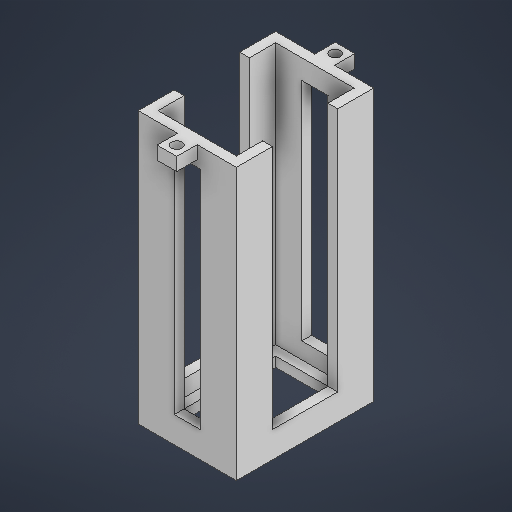
# Autodesk Inventor part: mocowanie-bateria
Saved by Autodesk Inventor 2026.2 (Build 302298010, 298A)
## iProperties
Created: 2026-04-20
Part Number: mocowanie-bateria
Material: Ogólny
Document SubType Name: Modeling
Designer: macie
Density: 1 g/cm^3
Appearance: Domyślna
Author: macie
Autodesk Inventor part; units mm, degrees
ref_plane "YZ Plane" through (0, 0, 0) normal (1, 0, 0) x (0, 1, 0)
ref_plane "XZ Plane" through (0, 0, 0) normal (0, 1, 0) x (-1, 0, 0)
ref_plane "XY Plane" through (0, 0, 0) normal (0, 0, 1) x (1, 0, 0)
sketch "Szkic1" plane through (0, 0, 0) normal (0, 1, 0) x (-1, 0, 0)
  line L0 (12, 18) -> (-12, 18)
  line L1 (-12, 18) -> (-12, -18)
  line L2 (-12, -18) -> (12, -18)
  line L3 (12, -18) -> (12, 18)
  line L4 (12, 18) -> (-12, -18) construction
  line L5 (-12, 18) -> (12, -18) construction
  line L6 (15, 21) -> (-15, 21)
  line L7 (-15, 21) -> (-15, -21)
  line L8 (-15, -21) -> (15, -21)
  line L9 (15, -21) -> (15, 21)
  line L10 (15, 21) -> (-15, -21) construction
  line L11 (-15, 21) -> (15, -21) construction
  line L12 (9, 15) -> (-9, 15)
  line L13 (-9, 15) -> (-9, -15)
  line L14 (-9, -15) -> (9, -15)
  line L15 (9, -15) -> (9, 15)
  line L16 (9, 15) -> (-9, -15) construction
  line L17 (-9, 15) -> (9, -15) construction
  point P0 (0, 0)
  dimension "d0" = 24
  dimension "d1" = 36
  dimension "d2" = 42
  dimension "d3" = 30
  dimension "d4" = 18
  dimension "d5" = 30
  constraints: 36 end point, 6 midpoint, 6 parallel, 3 horizontal, 3 perpendicular
  measures "d0" distance between parallel lines of L1 L3
  measures "d1" distance between parallel lines of L2 L0
  measures "d2" distance between parallel lines of L8 L6
  measures "d3" distance between parallel lines of L7 L9
  measures "d4" distance between parallel lines of L13 L15
  measures "d5" distance between parallel lines of L14 L12
extrude "Wyciągnięcie proste1" add sketch "Szkic1" along normal blind 3 contours L3 L2 L1 L0
extrude "Wyciągnięcie proste2" add sketch "Szkic1" along normal blind 8 contours L9 L8 L7 L6
sketch "Szkic2" plane through (0, 8, 0) normal (0, 1, 0) x (1, 0, 0)
  line L0 (-15, 21) -> (-15, -21) projected
  line L1 (-12, -18) -> (12, -18) projected
  line L2 (-15, -21) -> (-4, -21)
  line L3 (-4, -21) -> (-4, -18)
  line L4 (-4, -18) -> (-15, -18)
  line L5 (-15, -18) -> (-15, -21)
  line L6 (-12, -18) -> (-15, -18)
  line L7 (-15, -18) -> (-15, -10)
  line L8 (-15, -10) -> (-12, -10)
  line L9 (-12, -10) -> (-12, -18)
  line L10 (-15, -21) -> (-15, -10)
  line L11 (0, 0) -> (-18.1992, 0)
  line L12 (-15, 21) -> (-4, 21)
  line L13 (-4, 21) -> (-4, 18)
  line L14 (-4, 18) -> (-15, 18)
  line L15 (-15, 10) -> (-12, 10)
  line L16 (-12, 10) -> (-12, 18)
  line L17 (4, 18) -> (15, 18)
  line L18 (4, 21) -> (4, 18)
  line L19 (15, 21) -> (4, 21)
  line L20 (15, 21) -> (15, 10)
  line L21 (15, 10) -> (12, 10)
  line L22 (12, 10) -> (12, 18)
  line L23 (12, -10) -> (12, -18)
  line L24 (15, -10) -> (12, -10)
  line L25 (4, -18) -> (15, -18)
  line L26 (15, -21) -> (4, -21)
  line L27 (4, -21) -> (4, -18)
  line L28 (15, -21) -> (15, 21) projected
  line L29 (15, -21) -> (15, -10)
  point P0 (-4, -19.5)
  point P1 (4, 19.5)
  dimension "d10" = 11
  dimension "d11" = 8
  dimension "d12" = 18.1992
  dimension "d15" = 360
  constraints: 54 end point, 6 symmetric about line, 4 parallel, 3 horizontal, 2 collinear, 2 perpendicular, 2 point on line, 1 midpoint, 53 other
  measures "d10" distance from line of L0 point (-4, -19.5)
  measures "d11" distance between parallel lines of L8 L4
  measures "d12" distance of L11.start L11.end
extrude "Wyciągnięcie proste3" add sketch "Szkic2" along normal blind 75
sketch "Szkic3" plane through (-4, 8, 21) normal (1, 0, 0) x (0, 0, -1)
  line L0 (0, 75) -> (3, 75) projected
  line L1 (3, -5) -> (3, 75) projected
  line L2 (0, 75) -> (3, 75)
  line L3 (3, 75) -> (3, 69)
  line L4 (3, 69) -> (0, 69)
  line L5 (0, 69) -> (0, 75)
  line L6 (21, 73.1209) -> (21, -14.9491)
  line L7 (0, -8) -> (0, 75) projected
  line L8 (42, 75) -> (39, 75)
  line L9 (39, -5) -> (39, 75)
  line L10 (39, 69) -> (42, 69)
  line L11 (42, 69) -> (42, 75)
  point P0 (21, -8)
  dimension "d19" = 6
  dimension "d20" = 88.0699
  dimension "d21" = 21
  constraints: 18 end point, 5 symmetric about line, 2 parallel, 2 point on line, 1 horizontal, 1 perpendicular, 1 vertical
  measures "d19" distance between parallel lines of L4 L0
  measures "d20" distance of L6.end L6.start
  measures "d21" distance between parallel lines of L7 L6
extrude "Wyciągnięcie proste4" add sketch "Szkic3" along normal blind 9
sketch "Szkic7" plane through (-15, 0, 21) normal (0, 0, 1) x (1, 0, 0)
  line L0 (27, 83) -> (3, 83) projected
  line L1 (12, 83) -> (18, 83)
  line L2 (18, 83) -> (18, 79)
  line L3 (18, 79) -> (12, 79)
  line L4 (12, 79) -> (12, 83)
  line L5 (19, 8) -> (19, 77) projected
  point P0 (15, 0)
  point P1 (18, 81)
  dimension "d29" = 6
  dimension "d30" = 1
  dimension "d31" = 4
  constraints: 8 end point, 2 parallel, 1 horizontal, 1 midpoint, 1 perpendicular, 1 point on line
  measures "d29" distance between parallel lines of L2 L4
  measures "d30" distance from line of L5 point (18, 81)
  measures "d31" distance between parallel lines of L0 L3
extrude "Wyciągnięcie proste6" add sketch "Szkic7" along normal blind 6.25
mirror "Odbij1" about plane through (0, 0, 0) normal (0, 0, 1) of "Wyciągnięcie proste6"
sketch "Szkic8" plane through (0, 83, 0) normal (0, 1, 0) x (1, 0, 0)
  line L0 (3, -27.25) -> (-3, -27.25) projected
  line L1 (-3, -21) -> (-3, -27.25) projected
  point P0 (0, 0)
  point P1 (0, -24.25)
  dimension "d34" = 3
  dimension "d35" = 3
  measures "d34" distance from line of L0 point (0, -24.25)
  measures "d35" distance from line of point (0, -24.25) L1
hole "Otwór1" at (0, 83, 24.25) direction (0, -1, 0) diameter 3.2 end through all
mirror "Odbij2" about plane through (0, 0, 0) normal (0, 0, 1) of "Otwór1"
